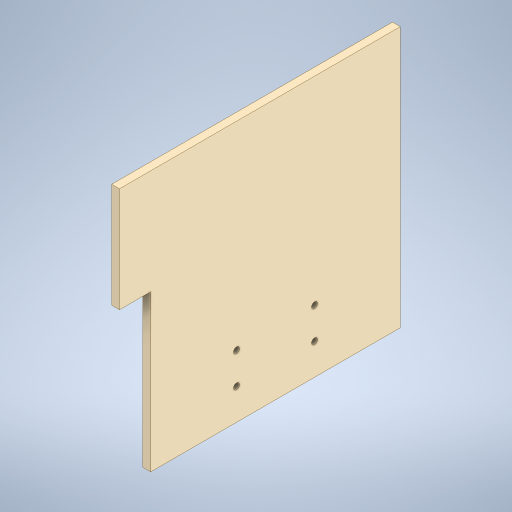
# Autodesk Inventor part: Wood-7
Saved by Autodesk Inventor 2024 (Build 280153000, 153)
## iProperties
Created: 2024-03-20
Part Number: Wood-7
Material: Generic
Document SubType Name: Modeling
Designer: Liz
Density: 1 g/cm^3
Appearance: Default
Author: Liz
Autodesk Inventor part; units mm, degrees
ref_plane "YZ Plane" through (0, 0, 0) normal (1, 0, 0) x (0, 1, 0)
ref_plane "XZ Plane" through (0, 0, 0) normal (0, 1, 0) x (-1, 0, 0)
ref_plane "XY Plane" through (0, 0, 0) normal (0, 0, 1) x (1, 0, 0)
sketch "Sketch1" plane through (0, 0, 0) normal (1, 0, 0) x (0, 1, 0)
  line L0 (-212.25, 203.2) -> (212.25, 203.2)
  line L1 (212.25, 203.2) -> (212.25, -203.2)
  line L2 (212.25, -203.2) -> (-212.25, -203.2)
  line L3 (-212.25, -203.2) -> (-212.25, 203.2)
  line L4 (-212.25, 203.2) -> (212.25, -203.2) construction
  line L5 (212.25, 203.2) -> (-212.25, -203.2) construction
  point P0 (0, 0)
  dimension "d0" = 406.4
  dimension "d1" = 424.5
  constraints: 12 end point, 2 midpoint, 2 parallel, 1 horizontal, 1 perpendicular
  measures "d0" distance of L2.end L0.start
  measures "d1" distance of L0.start L0.end
extrude "Extrusion1" add sketch "Sketch1" along normal mid plane 12.7
sketch "Sketch2" plane through (6.35, 0, 0) normal (1, 0, 0) x (0, 0, -1)
  circle A0 centre (-63.5, -161.45) radius 5
  line L0 (203.2, -212.25) -> (203.2, 212.25) projected
  line L1 (203.2, 212.25) -> (-203.2, 212.25) projected
  line L2 (-203.2, 212.25) -> (-203.2, -212.25) projected
  line L3 (-203.2, -212.25) -> (203.2, -212.25) projected
  circle A1 centre (63.5, -161.45) radius 5
  circle A2 centre (-63.5, -110.65) radius 5
  circle A3 centre (63.5, -110.65) radius 5
  point P0 (0, 0)
  dimension "d6" = 127
  dimension "d9" = 50.8
  dimension "d12" = 10
  dimension "d14" = 63.5
  dimension "d15" = 50.8
  constraints: 4 centre point, 1 horizontal, 1 vertical, 6 other
  measures "d6" distance of A0.centre A1.centre
  measures "d9" distance of A0.centre A2.centre
  measures "d12" diameter of A0
  measures "d14" horizontal distance of point (0, 0) A0.centre
  measures "d15" distance from line of L3 A0.centre
extrude "Extrusion2" cut sketch "Sketch2" against normal blind 12.7 contours A0 | A1 | A2 | A3
sketch "Sketch3" plane through (-6.35, -212.25, 203.2) normal (0, 0, 1) x (1, 0, 0)
  line L0 (0, 424.5) -> (12.7, 424.5) projected
  line L1 (12.7, 0) -> (12.7, 424.5) projected
  line L2 (0, 424.5) -> (12.7, 424.5)
  line L3 (12.7, 424.5) -> (12.7, 254)
  line L4 (12.7, 254) -> (0, 254)
  line L5 (0, 254) -> (0, 424.5)
  point P0 (6.35, 212.25)
  dimension "d20" = 170.5
  constraints: 8 end point, 2 parallel, 1 horizontal, 1 perpendicular, 1 point on line
  measures "d20" distance of L4.end L0.start
extrude "Extrusion3" add sketch "Sketch3" along normal blind 50.8
body "Solid1"
